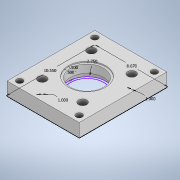
# Autodesk Inventor part: Wash_Base_Bottom
Saved by Autodesk Inventor 2022 (Build 260153000, 153)
## iProperties
Created: 2021-10-22
Part Number: Wash_Base_Bottom
Material: Generic
Document SubType Name: Modeling
Designer: tgr41
Density: 1 g/cm^3
Appearance: Default
Author: tgr41
Autodesk Inventor part; units mm, degrees
ref_plane "YZ Plane" through (0, 0, 0) normal (1, 0, 0) x (0, 1, 0)
ref_plane "XZ Plane" through (0, 0, 0) normal (0, 1, 0) x (-1, 0, 0)
ref_plane "XY Plane" through (0, 0, 0) normal (0, 0, 1) x (1, 0, 0)
sketch "Sketch1" plane through (0, 0, 0) normal (0, 1, 0) x (-1, 0, 0)
  line L0 (0, 0) -> (220.218, 0)
  line L1 (220.218, 0) -> (220.218, -267.97)
  line L2 (220.218, -267.97) -> (0, -267.97)
  line L3 (0, -267.97) -> (0, 0)
  circle A0 centre (110.109, -133.985) radius 57.15
  circle A1 centre (110.109, -133.985) radius 50.8
  line L4 (220.218, 0) -> (220.218, -25.4)
  circle A2 centre (201.168, -248.92) radius 9.525
  circle A3 centre (201.168, -19.05) radius 9.525
  circle A4 centre (19.05, -248.92) radius 9.525
  circle A5 centre (19.05, -19.05) radius 9.525
  line L5 (181.0385, -172.085) -> (193.7385, -172.085)
  line L6 (193.7385, -172.085) -> (206.4385, -172.085)
  line L7 (181.0385, -172.085) -> (206.4385, -172.085)
  line L8 (206.4385, -172.085) -> (206.4385, -159.385)
  line L9 (206.4385, -159.385) -> (181.0385, -159.385)
  line L10 (181.0385, -95.885) -> (193.7385, -95.885)
  line L11 (193.7385, -95.885) -> (206.4385, -95.885)
  line L12 (181.0385, -95.885) -> (206.4385, -95.885)
  line L13 (206.4385, -95.885) -> (206.4385, -108.585)
  line L14 (206.4385, -108.585) -> (181.0385, -108.585)
  line L15 (181.0385, -172.085) -> (181.0385, -159.385)
  line L16 (181.0385, -108.585) -> (181.0385, -95.885)
  circle A6 centre (171.8873, -209.1593) radius 34.925
  circle A7 centre (48.3307, -209.1593) radius 34.925
  circle A8 centre (171.8873, -58.8107) radius 34.925
  circle A9 centre (48.3307, -58.8107) radius 34.925
  circle A10 centre (171.8873, -58.8107) radius 12.7
  circle A11 centre (171.8873, -209.1593) radius 12.7
  circle A12 centre (48.3307, -209.1593) radius 12.7
  circle A13 centre (48.3307, -58.8107) radius 12.7
  dimension "d0" = 220.218
  dimension "d1" = 267.97
  dimension "d41" = 12.7
  dimension "d44" = 12.7
  dimension "d52" = 69.85
  dimension "d53" = 25.4
  dimension "d54" = 25.4
  constraints: 34 end point, 14 centre point, 5 coincident, 4 perpendicular, 3 equal length, 3 point on line, 2 horizontal, 1 vertical, 1 other
  measures "d0" distance of L1.end L2.end
  measures "d1" distance of L0.end L1.end
  measures "d41" distance of L5.end L5.start
  measures "d44" distance of L6.end L8.end
  measures "d52" diameter of A6
  measures "d53" diameter of A10
  measures "d54" diameter of A12
extrude "Extrusion3" add sketch "Sketch1" along normal blind 40.64 contours L0 L1 L2 L3 | A0 | A1 | A2 | A3 | A4 | A5 | L15 L9 L8 L6 L5 | L10 L11 L13 L14 L16 | A6 | A7 | A8 | A9 | A10 | A11 | A12 | A13
extrude "Extrusion4" cut sketch "Sketch1" along normal blind 40.64 contours A1
extrude "Extrusion5" cut sketch "Sketch1" along normal blind 12.7 contours A0 | A1
sketch "Sketch3" plane through (0, 40.64, 0) normal (0, 1, 0) x (1, 0, 0)
  line L0 (0, 267.97) -> (-220.218, 267.97) projected
  line L1 (-220.218, 0) -> (0, 0) projected
  circle A0 centre (-110.109, 133.985) radius 57.15
  dimension "d21" = 114.3
  constraints: 1 centre point
  measures "d21" diameter of A0
extrude "Extrusion6" cut sketch "Sketch3" against normal blind 3.175
extrude "Extrusion8" cut sketch "Sketch1" along normal blind 87.3125 contours A2 | A3 | A4 | A5
extrude "Extrusion9" add sketch "Sketch1" against normal blind 25.4 contours L15 L9 L8 L6 L5 | L10 L11 L13 L14 L16
fillet "Fillet1" radius 12.7 4 edges at (-181.0385, -25.4, -102.235) (-181.0385, -25.4, -165.735) (-206.4385, -25.4, -165.735) (-206.4385, -25.4, -102.235)
sketch "Sketch4" plane through (-206.4385, 0, -95.885) normal (0, 0, 1) x (1, 0, 0)
  arc A0 (0, -12.7) -> (25.4, -12.7) centre (12.7, -12.7) ccw projected
  circle A1 centre (12.7, -12.7) radius 6.35
  point P0 (206.4385, 0)
  dimension "d48" = 12.7
  constraints: 1 centre point, 1 coincident
  measures "d48" diameter of A1
extrude "Extrusion10" cut sketch "Sketch4" along normal mid plane 436.5625
extrude "Extrusion11" cut sketch "Sketch1" along normal blind 125.4125 contours A10 | A11 | A12 | A13
body "Solid3"
